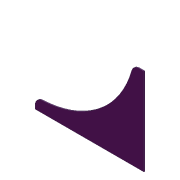
# Autodesk Inventor part: Shovel_SideWall
Saved by Autodesk Inventor 2012 (Build 160160000, 160)
## iProperties
Created: 2013-01-29
Part Number: Shovel_SideWall
Material: Aluminum-6061
Document SubType Name: Modeling
Designer: JesseK
Density: 2.71 g/cm^3
Mass: 50.5348 g
Surface Area: 244.583 cm^2
Volume: 18.6475 cm^3
Author: JesseK
Autodesk Inventor part; units mm, degrees
ref_plane "YZ Plane" through (0, 0, 0) normal (1, 0, 0) x (0, 1, 0)
ref_plane "XZ Plane" through (0, 0, 0) normal (0, 1, 0) x (-1, 0, 0)
ref_plane "XY Plane" through (0, 0, 0) normal (0, 0, 1) x (1, 0, 0)
sketch "Sketch1" plane through (0, 0, 0) normal (0, 0, 1) x (1, 0, 0)
  line L0 (-109.0864, -41.6468) -> (-109.0864, -22.5968)
  line L1 (62.3636, 110.7532) -> (81.4136, 110.7532)
  line L2 (81.4136, 110.7532) -> (81.4136, -41.6468)
  line L3 (81.4136, -41.6468) -> (-109.0864, -41.6468)
  arc A0 (-109.0864, -22.5968) -> (62.3636, 110.7532) centre (-104.0104, 147.7699) ccw
  point P0 (0, 0)
  dimension "d0" = 19.05
  dimension "d1" = 152.4
  dimension "d2" = 19.05
  dimension "d3" = 190.5
  constraints: 8 end point, 2 horizontal, 2 point on circle, 2 vertical, 1 centre point
  measures "d0" distance of L0.start L0.end
  measures "d1" distance of L1.end L2.end
  measures "d2" distance of L1.start L1.end
  measures "d3" distance of L2.end L0.start
extrude "Extrusion1" add sketch "Sketch1" along normal blind 1.5875
fillet "Fillet1" radius 12.7 2 edges at (62.3636, 110.7532, 0.7937) (-109.0864, -22.5968, 0.7937)
body "Solid1"
